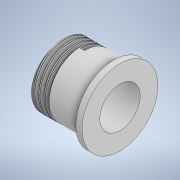
# Autodesk Inventor part: pipeForFrontPipeDrain
Saved by Autodesk Inventor 2021.1 (Build 251245010, 245A)
## iProperties
Created: 2020-10-20
Part Number: pipeForFrontPipeDrain
Material: Generic
Document SubType Name: Modeling
Designer: robst
Density: 1 g/cm^3
Appearance: Default
Author: robst
Autodesk Inventor part; units mm, degrees
ref_plane "YZ Plane" through (0, 0, 0) normal (1, 0, 0) x (0, 1, 0)
ref_plane "XZ Plane" through (0, 0, 0) normal (0, 1, 0) x (-1, 0, 0)
ref_plane "XY Plane" through (0, 0, 0) normal (0, 0, 1) x (1, 0, 0)
sketch "Sketch2" plane through (0, 0, 0) normal (0, 0, 1) x (1, 0, 0)
  line L0 (0, 0) -> (0, 18.415)
  line L1 (0, 18.415) -> (-2.9977, 18.415)
  line L2 (-2.9977, 18.415) -> (-2.9977, 15.24)
  line L3 (-2.9977, 15.24) -> (-22.0477, 15.24)
  line L4 (-22.0477, 15.24) -> (-22.0477, 9.815)
  line L5 (-22.0477, 9.815) -> (0, 9.815)
  line L6 (-34.0773, 0) -> (5.6795, 0) projected
  line L7 (-22.0477, 9.815) -> (-28.3977, 9.815)
  line L8 (-28.3977, 9.815) -> (-28.3977, 15.24)
  line L9 (-28.3977, 15.24) -> (-22.0477, 15.24)
  line L10 (-22.0477, 15.24) -> (-22.0477, 9.815)
  dimension "d0" = 18.415
  dimension "d1" = 9.815
  dimension "d2" = 2.9977
  dimension "d3" = 19.05
  dimension "d5" = 15.24
  dimension "d6" = 6.35
  constraints: 20 end point, 6 perpendicular, 2 parallel, 1 collinear, 1 horizontal, 1 point on line, 1 vertical
  measures "d0" distance from line of L0.start L1
  measures "d1" distance from line of L5 L0.start
  measures "d2" distance between parallel lines of L0 L2
  measures "d3" distance from line of L3.end L2
  measures "d5" distance from line of L3 L0.start
  measures "d6" distance between parallel lines of L8 L4
revolve "Revolution1" add sketch "Sketch2" angle 360 about axis through (-10, 0, 0) along (1, 0, 0)
sketch "Sketch4" plane through (0, 0, 0) normal (0, 0, 1) x (1, 0, 0)
  line L0 (-31.8854, 15.1606) -> (-31.1511, 13.8887)
  line L1 (-30.7244, 13.8887) -> (-29.9901, 15.1606)
  arc A0 (-31.1511, 13.8887) -> (-30.7244, 13.8887) centre (-30.9377, 14.0119) ccw
  line L2 (-32.5301, 15.1606) -> (-33.8011, 12.9592)
  line L3 (-29.3454, 15.1606) -> (-28.8919, 14.375)
  arc A1 (-31.8854, 15.1606) -> (-32.5301, 15.1606) centre (-32.2077, 14.9745) ccw
  arc A2 (-29.3454, 15.1606) -> (-29.9901, 15.1606) centre (-29.6677, 14.9745) ccw
  line L4 (-32.2077, 15.3467) -> (-29.6677, 15.3467)
  line L5 (-28.3977, -15.24) -> (-28.3977, 15.24) construction
  line L6 (-28.3977, 0) -> (-33.4777, 0) construction
  line L7 (-33.8011, 12.9592) -> (-33.8011, 16.2117) construction
  point P0 (0, 0)
  dimension "d10" = 60
  dimension "d11" = 0.2464
  dimension "d12" = 60
  dimension "d13" = 60
  dimension "d15" = 2.54
  dimension "d16" = 5.08
  dimension "d17" = 1.27
  dimension "d18" = 15.3467
  dimension "d19" = 13.7655
  dimension "d20" = 30
  constraints: 14 end point, 8 point on circle, 6 tangent, 3 centre point, 2 horizontal, 1 equal radius, 1 midpoint, 1 vertical
  measures "d10" angle of L1 L0
  measures "d11" radius of A0
  measures "d12" angle of L0 L2
  measures "d13" angle of L3 L1
  measures "d15" distance of A2.centre A1.centre
  measures "d16" distance from line of L6.end L5
  measures "d17" distance from line of A2.centre L5
  measures "d18" distance between parallel lines of L4 L6
  measures "d19" distance edge to line of A0 L6
  measures "d20" angle of L7 L2
coil "Coil1" sketch "Sketch4" operation cut axis through (-10, 0, 0) along (1, 0, 0) pitch 2.54 turns 5 hand right
equation "\"d0\" = outsideRadius"
equation "\"d3\" = houseWallThickness"
equation "\"d5\" = holeRadius"
equation "\"d6\" = allowanceForThreadRing"
equation "\"d10\" = threadAngle"
equation "\"d11\" = a1RootRadius"
equation "\"d12\" = threadAngle"
equation "\"d13\" = threadAngle"
equation "\"d15\" = pitch"
equation "\"d16\" = 2 * pitch"
equation "\"d17\" = 0.5 * pitch"
equation "\"d18\" = 0.5 * a1MajorDiameter"
equation "\"d19\" = 0.5 * a1MinorDiameter"
equation "\"d20\" = 0.5 * threadAngle"
equation "\"d21\" = pitch"
equation "\"d22\" = threadDepth"
equation "\"holeDiameter\" = 30.48"
equation "\"pipeDiameter\" = 27.94"
equation "\"holeRadius\" = 0.5 * holeDiameter"
equation "\"pipeRadius\" = 0.5 * pipeDiameter"
equation "\"wallThickness\" = 3.175"
equation "\"houseWallThickness\" = 19.05"
equation "\"allowanceForThreadRing\" = 6.35"
equation "\"threadDepth\" = 12.7"
equation "\"outsideRadius\" = 0.5 * outsideDiameter"
equation "\"a1MajorDiameter\" = 30.69336"
equation "\"a1MinorDiameter\" = 27.53106"
equation "\"a1RootRadius\" = 0.24638"
equation "\"threadAngle\" = 60deg"
equation "\"pitch\" = 2.54"
equation "\"outsideDiameter\" = 36.83"
body "Solid1"
